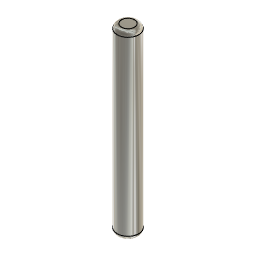
MG996R_Pin_Long v3 (Autodesk Fusion 360 design; units mm, degrees)
Autodesk Fusion 360 part; units mm, degrees
sketch "Sketch1" plane through (0, 0, 0) normal (0, 0, 1) x (1, 0, 0)
  circle A0 centre (0, 0) radius 0.75
  dimension "d1" = 1.5
  constraint coincident A0.centre origin
  measures "d1" diameter of A0
extrude "Extrude1" add sketch "Sketch1" along normal blind 12.5
fillet "Fillet1" radius 0.3 2 edges at (-0.6992, -0.2712, 12.5) (-0.6992, -0.2712, 0)
